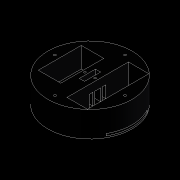
# Autodesk Inventor part: MainMiddle
Saved by Autodesk Inventor 2022 (Build 260153000, 153)
## iProperties
Created: 2020-12-05
Part Number: MainMiddle
Material: Generic
Document SubType Name: Modeling
Designer: Esketitttttt
Density: 1 g/cm^3
Appearance: Smooth - Black
Author: Esketitttttt
Autodesk Inventor part; units mm, degrees
ref_plane "Work Plane2" through (9.55, 10.6, 38.1) normal (0.8357, -0.5492, 0) x (0, 0, -1)
ref_plane "YZ Plane" through (0, 0, 0) normal (1, 0, 0) x (0, 1, 0)
ref_plane "XZ Plane" through (0, 0, 0) normal (0, 1, 0) x (-1, 0, 0)
sketch "Sketch1" plane through (0, 0, 0) normal (0, 1, 0) x (-1, 0, 0)
  line L0 (9.55, 26.67) -> (37.49, 26.67)
  line L1 (37.49, 26.67) -> (37.49, -26.67)
  line L2 (37.49, -26.67) -> (9.55, -26.67)
  line L3 (9.55, -26.67) -> (9.55, 26.67)
  line L4 (-9.55, 31.75) -> (-34.95, 31.75)
  line L5 (-34.95, 31.75) -> (-34.95, -31.75)
  line L6 (-34.95, -31.75) -> (-9.55, -31.75)
  line L7 (-9.55, -31.75) -> (-9.55, 31.75)
  line L8 (-9.55, -31.75) -> (-34.95, -31.75)
  line L9 (-34.95, -31.75) -> (-34.95, -38.1)
  line L10 (-34.95, -38.1) -> (-9.55, -38.1)
  line L11 (-9.55, -38.1) -> (-9.55, -31.75)
  line L12 (-34.95, 31.75) -> (-9.55, 31.75)
  line L13 (-9.55, 31.75) -> (-9.55, 38.1)
  line L14 (-9.55, 38.1) -> (-34.95, 38.1)
  line L15 (-34.95, 38.1) -> (-34.95, 31.75)
  line L16 (3.2, 10) -> (-3.2, 10)
  line L17 (-3.2, 10) -> (-3.2, -10)
  line L18 (-3.2, -10) -> (3.2, -10)
  line L19 (3.2, -10) -> (3.2, 10)
  line L20 (0, 10) -> (0, 0) construction
  line L21 (9.55, -26.67) -> (37.49, 26.67) construction
  line L22 (9.55, 26.67) -> (37.49, -26.67) construction
  line L23 (23.52, 26.67) -> (23.52, 0) construction
  line L24 (-9.55, 0) -> (-75.4632, 0) construction
  circle A0 centre (0, 0) radius 52.07
  dimension "d0" = 27.94
  dimension "d1" = 53.34
  dimension "d2" = 25.4
  dimension "d3" = 63.5
  dimension "d4" = 6.35
  dimension "d5" = 6.35
  dimension "d6" = 6.4
  dimension "d7" = 20
  dimension "d8" = 0
  dimension "d9" = 6.35
  dimension "d10" = 0
  dimension "d11" = 6.35
  dimension "d12" = 104.14
  constraints: 50 end point, 10 parallel, 7 horizontal, 5 perpendicular, 4 midpoint, 2 point on line, 2 vertical, 1 centre point, 1 coincident
  measures "d0" distance of L1.end L2.end
  measures "d1" distance of L0.end L1.end
  measures "d2" distance of L6.end L5.end
  measures "d3" distance of L5.end L4.end
  measures "d4" distance of L9.end L8.end
  measures "d5" distance of L13.end L12.end
  measures "d6" distance of L18.end L17.end
  measures "d7" distance of L17.end L16.end
  measures "d8" vertical distance of L23.end point (0, 0)
  measures "d9" distance between parallel lines of L19 L3
  measures "d10" vertical distance of point (0, 0) L24.end
  measures "d11" distance between parallel lines of L17 L7
  measures "d12" diameter of A0
extrude "Height for limitswitch to connectors" add sketch "Sketch1" along normal blind 10.6
sketch "Sketch2" plane through (0, 0, 0) normal (0, -1, 0) x (1, 0, 0)
  line L0 (3.2, -10) -> (3.2, 10) projected
  line L1 (3.2, 10) -> (-3.2, 10) projected
  line L2 (-3.2, 10) -> (-3.2, -10) projected
  line L3 (-3.2, -10) -> (3.2, -10) projected
  line L4 (3.2, 10) -> (3.2, 4.7) construction
  line L5 (3.2, -10) -> (3.2, 10) construction
  line L6 (3.2, 4.7) -> (3.2, -4.8) construction
  line L7 (-3.2, 10) -> (-3.2, -10) projected
  line L8 (3.2, -4.8) -> (-3.2, -4.8) construction
  line L9 (-3.2, -4.8) -> (-3.2, -6.07)
  line L10 (-3.2, -6.07) -> (3.2, -6.07)
  line L11 (3.2, -6.07) -> (3.2, -4.8)
  line L12 (-3.2, -6.07) -> (3.2, -6.07)
  line L13 (3.2, -6.07) -> (3.2, -3.53)
  line L14 (3.2, -3.53) -> (-3.2, -3.53)
  line L15 (-3.2, -3.53) -> (-3.2, -6.07)
  line L16 (3.2, 4.7) -> (-3.2, 4.7) construction
  line L17 (-3.2, 4.7) -> (-3.2, 3.43)
  line L18 (-3.2, 3.43) -> (3.2, 3.43)
  line L19 (3.2, 3.43) -> (3.2, 4.7)
  line L20 (-3.2, 3.43) -> (3.2, 3.43)
  line L21 (3.2, 3.43) -> (3.2, 5.97)
  line L22 (3.2, 5.97) -> (-3.2, 5.97)
  line L23 (-3.2, 5.97) -> (-3.2, 3.43)
  circle A0 centre (0, 0) radius 52.07 projected
  line L24 (-3.2, 10) -> (-3.2, -10) projected
  line L25 (3.2, 10) -> (-3.2, 10) projected
  line L26 (3.2, -10) -> (3.2, 10) projected
  line L27 (-3.2, -10) -> (3.2, -10) projected
  line L28 (-9.55, 26.67) -> (-37.49, 26.67) projected
  line L29 (-9.55, -26.67) -> (-9.55, 26.67) projected
  line L30 (-37.49, -26.67) -> (-9.55, -26.67) projected
  line L31 (-37.49, 26.67) -> (-37.49, -26.67) projected
  line L32 (34.95, -38.1) -> (34.95, 38.1) projected
  line L33 (9.55, -38.1) -> (34.95, -38.1) projected
  line L34 (9.55, 38.1) -> (9.55, -38.1) projected
  line L35 (34.95, 38.1) -> (9.55, 38.1) projected
  line L36 (9.55, 38.1) -> (9.55, -38.1) projected
  line L37 (3.2, 10) -> (9.55, 10)
  line L38 (9.55, 10) -> (9.55, 5.97)
  line L39 (9.55, 5.97) -> (3.2, 5.97)
  line L40 (3.2, 5.97) -> (3.2, 10)
  line L41 (3.2, 3.43) -> (9.55, 3.43)
  line L42 (9.55, 3.43) -> (9.55, -3.53)
  line L43 (9.55, -3.53) -> (3.2, -3.53)
  line L44 (3.2, -3.53) -> (3.2, 3.43)
  line L45 (-9.55, -26.67) -> (-9.55, 26.67) projected
  line L46 (-3.2, 10) -> (-9.55, 10)
  line L47 (-9.55, 10) -> (-9.55, 5.97)
  line L48 (-9.55, 5.97) -> (-3.2, 5.97)
  line L49 (-3.2, 5.97) -> (-3.2, 10)
  line L50 (-3.2, 3.43) -> (-9.55, 3.43)
  line L51 (-9.55, 3.43) -> (-9.55, -3.53)
  line L52 (-9.55, -3.53) -> (-3.2, -3.53)
  line L53 (-3.2, -3.53) -> (-3.2, 3.43)
  line L54 (3.2, -6.07) -> (9.55, -6.07)
  line L55 (9.55, -6.07) -> (9.55, -10)
  line L56 (9.55, -10) -> (3.2, -10)
  line L57 (3.2, -10) -> (3.2, -6.07)
  line L58 (-3.2, -6.07) -> (-9.55, -6.07)
  line L59 (-9.55, -6.07) -> (-9.55, -10)
  line L60 (-9.55, -10) -> (-3.2, -10)
  line L61 (-3.2, -10) -> (-3.2, -6.07)
  point P0 (3.2, -6.07)
  point P1 (-3.2, -3.53)
  point P2 (3.2, 3.43)
  point P3 (3.2, 3.43)
  point P4 (-3.2, -3.53)
  point P5 (3.2, -6.07)
  dimension "d15" = 5.3
  dimension "d16" = 9.5
  dimension "d17" = 1.27
  dimension "d18" = 2.54
  dimension "d20" = 1.27
  dimension "d21" = 2.54
  constraints: 84 end point, 20 parallel, 13 point on line, 10 horizontal, 10 perpendicular
  measures "d15" distance of L0.end L4.end
  measures "d16" distance of L4.end L6.end
  measures "d17" distance of L9.end L8.end
  measures "d18" distance of L13.end L12.end
  measures "d20" distance of L17.end L17.start
  measures "d21" distance of L21.end L20.end
extrude "Extrusion2" add sketch "Sketch2" along normal blind 14.8 contours L10 L2 L14 L0 | L0 L43 L34 L54 | L58 L29 L52 L2 | L18 L2 L22 L0 | L0 L39 L34 L41 | L50 L29 L48 L2 | A0
sketch "Sketch6" plane through (0, 0, 0) normal (0, -1, 0) x (1, 0, 0)
  line L0 (9.55, 3.43) -> (3.2, 3.43) construction
  line L1 (3.2, -3.53) -> (3.2, 3.43) construction
  line L2 (3.2, -3.53) -> (9.55, -3.53) construction
  line L3 (9.55, 3.43) -> (9.55, -3.53) construction
  line L4 (-3.2, 3.43) -> (-9.55, 3.43) construction
  line L5 (-9.55, -3.53) -> (-9.55, 3.43) construction
  line L6 (-9.55, -3.53) -> (-3.2, -3.53) construction
  line L7 (-3.2, 3.43) -> (-3.2, -3.53) construction
  line L8 (-9.55, -3.53) -> (-3.2, 3.43) construction
  line L9 (-3.2, 3.43) -> (-9.55, 3.43) construction
  line L10 (-3.2, -3.53) -> (-9.55, 3.43) construction
  line L11 (9.55, 3.43) -> (9.55, -3.53) construction
  line L12 (9.55, 3.43) -> (3.2, -3.53) construction
  line L13 (3.2, -3.53) -> (9.55, -3.53) construction
  line L14 (9.55, 3.43) -> (3.2, 3.43) construction
  line L15 (9.55, -3.53) -> (3.2, 3.43) construction
  circle A0 centre (6.375, -0.05) radius 1.27
  circle A1 centre (-6.375, -0.05) radius 1.27
  point P0 (0, 0)
  dimension "d36" = 2.54
  dimension "d37" = 2.54
  constraints: 8 end point, 2 centre point, 2 midpoint
  measures "d36" diameter of A0
  measures "d37" diameter of A1
extrude "Extrusion4" cut sketch "Sketch6" against normal through all
sketch "Sketch7" plane through (0, -14.8, 0) normal (0, -1, 0) x (1, 0, 0)
  circle A0 centre (0, 0) radius 52.07 projected
  line L0 (-9.55, -26.67) -> (-37.49, -26.67) projected
  line L1 (-37.49, -26.67) -> (-37.49, 26.67) projected
  line L2 (-37.49, 26.67) -> (-9.55, 26.67) projected
  line L3 (-9.55, 26.67) -> (-9.55, 10) projected
  line L4 (-9.55, 10) -> (9.55, 10) projected
  line L5 (9.55, 10) -> (9.55, 38.1) projected
  line L6 (9.55, 38.1) -> (34.95, 38.1) projected
  line L7 (34.95, 38.1) -> (34.95, -38.1) projected
  line L8 (34.95, -38.1) -> (9.55, -38.1) projected
  line L9 (9.55, -38.1) -> (9.55, -10) projected
  line L10 (9.55, -10) -> (-9.55, -10) projected
  line L11 (-9.55, -10) -> (-9.55, -26.67) projected
extrude "Bottom" add sketch "Sketch7" along normal blind 6.35 contours A0 | L0 L1 L2 L3 L4 L5 L6 L7 L8 L9 L10 L11
sketch "Sketch8" plane through (9.55, 10.6, 38.1) normal (1, 0, 0) x (0, 0, -1)
  line L0 (11.43, -25.4) -> (28.1, -25.4) projected
  line L1 (28.1, -25.4) -> (0, -25.4) projected
  line L2 (0, -25.4) -> (76.2, -25.4) projected
  line L3 (76.2, -25.4) -> (48.1, -25.4) projected
  line L4 (48.1, -25.4) -> (64.77, -25.4) projected
  line L5 (64.77, -25.4) -> (11.43, -25.4) projected
  line L6 (44.17, -25.4) -> (41.63, -25.4) projected
  line L7 (41.63, -25.4) -> (44.17, -25.4) projected
  line L8 (34.67, -25.4) -> (32.13, -25.4) projected
  line L9 (32.13, -25.4) -> (34.67, -25.4) projected
  line L10 (-13.97, -31.75) -> (90.17, -31.75) projected
  line L11 (64.77, -25.4) -> (11.43, -25.4) construction
  line L12 (38.1, -25.4) -> (38.1, -28.575) construction
  line L13 (38.1, -28.575) -> (63.5, -28.575) construction
  line L14 (63.5, -28.575) -> (63.5, -27.305)
  line L15 (63.5, -27.305) -> (38.1, -27.305)
  line L16 (38.1, -27.305) -> (38.1, -28.575) construction
  line L17 (63.5, -27.305) -> (12.7, -27.305)
  line L18 (12.7, -27.305) -> (12.7, -29.845)
  line L19 (12.7, -29.845) -> (63.5, -29.845)
  line L20 (63.5, -29.845) -> (63.5, -27.305)
  point P0 (38.1, -10.6)
  dimension "d42" = 3.175
  dimension "d43" = 25.4
  dimension "d44" = 1.27
  dimension "d45" = 50.8
  dimension "d46" = 2.54
  constraints: 18 end point, 4 parallel, 2 horizontal, 2 perpendicular, 1 vertical, 2 other
  measures "d42" distance of L12.start L12.end
  measures "d43" distance of L15.end L14.end
  measures "d44" distance of L14.end L13.end
  measures "d45" distance of L19.end L18.end
  measures "d46" distance of L18.end L17.end
extrude "Extrusion6" cut sketch "Sketch8" along normal through all both and the other way through all
sketch "Sketch9" plane through (0, 10.6, 0) normal (0, 1, 0) x (1, 0, 0)
  line L0 (34.95, 38.1) -> (34.95, -38.1) construction
  line L1 (34.95, 0) -> (52.07, 0) construction
  circle A0 centre (0, 0) radius 52.07 construction
  circle A1 centre (-6.375, 0.05) radius 1.27 projected
  circle A2 centre (6.375, 0.05) radius 1.27 projected
  circle A3 centre (0, 0) radius 52.07 projected
  line L2 (-3.2, -10) -> (-3.2, 10) projected
  line L3 (-3.2, 10) -> (3.2, 10) projected
  line L4 (3.2, 10) -> (3.2, -10) projected
  line L5 (3.2, -10) -> (-3.2, -10) projected
  line L6 (-9.55, -26.67) -> (-37.49, -26.67) projected
  line L7 (-37.49, -26.67) -> (-37.49, 26.67) projected
  line L8 (-37.49, 26.67) -> (-9.55, 26.67) projected
  line L9 (-9.55, 26.67) -> (-9.55, -26.67) projected
  line L10 (34.95, 38.1) -> (34.95, -38.1) projected
  line L11 (34.95, -38.1) -> (9.55, -38.1) projected
  line L12 (9.55, -38.1) -> (9.55, 38.1) projected
  line L13 (9.55, 38.1) -> (34.95, 38.1) projected
  circle A4 centre (43.51, 0) radius 1.4
  circle A5 centre (0, 43.51) radius 1.4
  circle A6 centre (-43.51, 0) radius 1.4
  circle A7 centre (0, -43.51) radius 1.4
  dimension "d51" = 360
  dimension "d53" = 2.8
  dimension "d56" = 360
  dimension "d24" = 8.335
  dimension "d25" = 6.35
  dimension "d26" = 6.35
  dimension "d27" = 2.54
  dimension "d28" = 2.54
  dimension "d29" = 2.54
  dimension "d30" = 2.54
  constraints: 4 centre point, 2 end point, 2 midpoint, 1 coincident, 1 horizontal, 1 horizontal alignment, 15 other
  measures "d53" diameter of A4
extrude "Extrusion7" cut sketch "Sketch9" against normal blind 7.46 contours A4 | A5 | A6 | A7
ref_plane "Work Plane1" through (0, 10.6, 18.335) normal (0.5492, 0.8357, 0) x (0.8357, -0.5492, 0)
sketch "Sketch5" plane through (9.55, 10.6, 38.1) normal (0.8357, -0.5492, 0) x (0, 0, -1)
  ellipse E0 centre (19.765, -5.2444) end of major axis (21.035, -5.2444) minor radius 0.6974 projected
  ellipse E1 centre (56.435, -5.2444) end of major axis (57.705, -5.2444) minor radius 0.6974 projected
  point P0 (38.1, -14.1031)
body "Solid1"
